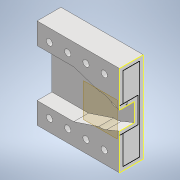
# Autodesk Inventor part: body
Saved by Autodesk Inventor 2022 (Build 260153000, 153)
## iProperties
Created: 2022-04-23
Part Number: body
Material: Generic
Document SubType Name: Modeling
Designer: efred
Density: 1 g/cm^3
Appearance: Default
Author: efred
Autodesk Inventor part; units mm, degrees
ref_plane "Work Plane1" through (0, 0, 0) normal (0, 0, 1) x (1, 0, 0)
sketch "Sketch1" plane through (0, 0, 0) normal (0, 0, 1) x (1, 0, 0)
  circle A0 centre (8, 0) radius 5 construction
  circle A1 centre (0, 18) radius 2 construction
  circle A2 centre (0, -18) radius 2 construction
  arc A3 (-10.2835, -9.5) -> (-3, -13.6748) centre (0, 0) ccw construction
  line L0 (-3, -13.6748) -> (-3, -18) construction
  arc A4 (-3, -18) -> (3, -18) centre (0, -18) ccw construction
  line L1 (3, -18) -> (3, -13.6748) construction
  arc A5 (3, -13.6748) -> (3, 13.6748) centre (0, 0) ccw construction
  line L2 (3, 13.6748) -> (3, 18) construction
  arc A6 (3, 18) -> (-3, 18) centre (0, 18) ccw construction
  line L3 (-3, 18) -> (-3, 13.6748) construction
  arc A7 (-3, 13.6748) -> (-10.2835, 9.5) centre (0, 0) ccw construction
  line L4 (-10.2835, 9.5) -> (-15.2835, 9.5) construction
  line L5 (-15.2835, 9.5) -> (-15.2835, -9.5) construction
  line L6 (-15.2835, -9.5) -> (-10.2835, -9.5) construction
  circle A8 centre (8, 0) radius 5.2
  circle A9 centre (0, -18) radius 1.7
  circle A10 centre (0, 18) radius 1.7
  line L7 (8, 0) -> (0, 0) construction
  line L8 (8, 0) -> (0, 0)
  line L9 (18.2, 24.7) -> (-6.7, 24.7)
  line L10 (-6.7, 24.7) -> (-6.7, -24.7)
  line L11 (-6.7, -24.7) -> (18.2, -24.7)
  line L12 (18.2, -24.7) -> (18.2, 24.7)
  point P0 (13.2, 0)
  point P1 (-1.7, 18)
  point P2 (0, 19.7)
  dimension "d0" = 0.2
  dimension "d3" = 5
  dimension "d4" = 5
  dimension "d5" = 5
  dimension "d20" = 3.4
  constraints: 12 end point, 3 equal length, 3 horizontal alignment, 2 centre point, 2 horizontal, 2 point on circle, 1 perpendicular, 1 vertical alignment, 4 other
  measures "d3" distance from line of point (13.2, 0) L12
  measures "d4" distance from line of L10 A10.start
  measures "d5" distance from line of A10.end L9
  measures "d20" diameter of A9
ref_plane "Work Plane2" through (3, -5, 1.9) normal (0, 0, 1) x (1, 0, 0)
ref_plane "Work Plane3" through (8, 0, 2) normal (0, 0, 1) x (1, 0, 0)
extrude "Extrusion1" add sketch "Sketch1" along normal up to surface (2 mm away)
sketch "Sketch2" plane through (-6.7, 24.7, 2) normal (0, 0, 1) x (1, 0, 0)
  circle A0 centre (6.7, -6.7) radius 1.7 projected
  circle A1 centre (6.7, -42.7) radius 1.7 projected
  circle A2 centre (14.7, -24.7) radius 5.2 construction
  line L0 (0, 0) -> (24.9, 0) projected
  line L1 (0, -49.4) -> (0, 0) projected
  line L2 (24.9, -49.4) -> (0, -49.4) projected
  line L3 (24.9, 0) -> (24.9, -49.4) projected
  circle A3 centre (14.7, -24.7) radius 2.5 construction
  circle A4 centre (14.7, -24.7) radius 2.7
  point P0 (6.7, -24.7)
  dimension "d8" = 0.2
  constraints: 1 centre point
  measures "d8" radial gap between concentric circles of A3 A4
ref_plane "Work Plane4" through (9.5, -2, 4.9) normal (0, 0, 1) x (1, 0, 0)
extrude "Extrusion2" add sketch "Sketch2" along normal up to surface (2.9 mm away)
sketch "Sketch3" plane through (-6.7, -24.7, 4.9) normal (0, 0, 1) x (1, 0, 0)
  arc A0 (18.0541, 25.7) -> (15.7, 28.0541) centre (14.7, 24.7) ccw construction
  line L0 (15.7, 33.0541) -> (15.7, 28.0541) construction
  line L1 (13.7, 33.0541) -> (15.7, 33.0541) construction
  line L2 (13.7, 28.0541) -> (13.7, 33.0541) construction
  arc A1 (13.7, 28.0541) -> (11.3459, 25.7) centre (14.7, 24.7) ccw construction
  line L3 (6.3459, 25.7) -> (11.3459, 25.7) construction
  line L4 (6.3459, 23.7) -> (6.3459, 25.7) construction
  line L5 (11.3459, 23.7) -> (6.3459, 23.7) construction
  arc A2 (11.3459, 23.7) -> (13.7, 21.3459) centre (14.7, 24.7) ccw construction
  line L6 (13.7, 16.3459) -> (13.7, 21.3459) construction
  line L7 (15.7, 16.3459) -> (13.7, 16.3459) construction
  line L8 (15.7, 21.3459) -> (15.7, 16.3459) construction
  arc A3 (15.7, 21.3459) -> (18.0541, 23.7) centre (14.7, 24.7) ccw construction
  line L9 (23.0541, 23.7) -> (18.0541, 23.7) construction
  line L10 (23.0541, 25.7) -> (23.0541, 23.7) construction
  line L11 (18.0541, 25.7) -> (23.0541, 25.7) construction
  circle A4 centre (14.7, 24.7) radius 8.4137 construction
  arc A5 (17.9486, 32.5696) -> (17.9486, 16.8304) centre (14.7, 24.7) ccw
  circle A6 centre (6.7, 42.7) radius 1.7 projected
  circle A7 centre (6.7, 6.7) radius 1.7 projected
  circle A8 centre (14.7, 24.7) radius 2.7 projected
  line L12 (0, 0) -> (0, 49.4) projected
  line L13 (24.9, 0) -> (0, 0) projected
  line L14 (24.9, 49.4) -> (24.9, 0) projected
  line L15 (0, 49.4) -> (24.9, 49.4) projected
  line L16 (0, 49.4) -> (0, 0) projected
  circle A9 centre (14.7, 24.7) radius 2.7 projected
  line L17 (14.7, 24.7) -> (0, 24.7) construction
  line L18 (17.9486, 16.8304) -> (24.9, 19.7)
  line L19 (24.9, 0) -> (24.9, 49.4) projected
  line L20 (17.9486, 32.5696) -> (24.9, 29.7)
  line L21 (13.7, 16.2452) -> (0, 11.7)
  line L22 (13.7, 33.1548) -> (0, 37.7)
  point P0 (6.7, 24.7)
  point P1 (0, 37.7)
  point P2 (24.9, 19.7)
  point P3 (0, 11.7)
  point P4 (0, 37.7)
  dimension "d11" = 0.1
  dimension "d13" = 10
  dimension "d17" = 5
  constraints: 10 end point, 3 point on circle, 3 point on line, 3 symmetric about line, 1 centre point, 1 coincident, 1 midpoint, 1 tangent, 1 vertical alignment, 4 other
  measures "d13" distance of L20.end L18.end
  measures "d17" vertical distance of L21.end A7.centre
ref_plane "Work Plane5" through (8, 0, 13.1) normal (0, 0, 1) x (-1, 0, 0)
ref_plane "Work Plane6" through (-0.3541, -8.3541, 13) normal (0, 0, 1) x (1, 0, 0)
extrude "Extrusion3" add sketch "Sketch3" along normal up to surface (8.1 mm away) contours A5 L22 L12 L15 L14 L20 | A5 L18 L14 L13 L12 L21
sketch "Sketch4" plane through (-6.7, -24.7, 0) normal (-1, 0, 0) x (0, 0, 1)
  line L0 (0, 49.4) -> (13, 49.4) projected
  line L1 (0, 49.4) -> (0, 0) projected
  line L2 (0, 0) -> (13, 0) projected
  line L3 (13, 0) -> (13, 11.7) projected
  line L4 (4.9, 11.7) -> (13, 11.7) projected
  line L5 (4.9, 11.7) -> (4.9, 37.7) projected
  line L6 (4.9, 37.7) -> (13, 37.7) projected
  line L7 (13, 37.7) -> (13, 49.4) projected
  point P0 (0, 24.7)
extrude "Extrusion4" add sketch "Sketch4" along normal blind 20
sketch "Sketch5" plane through (18.2, -24.7, 13) normal (0, 0, 1) x (1, 0, 0)
  circle A0 centre (-18.2, 6.7) radius 1.7 projected
  circle A1 centre (-18.2, 6.7) radius 1.7
  line L0 (0, 0) -> (-44.9, 0) projected
  circle A2 centre (-28.2, 6.7) radius 1.7
  circle A3 centre (-38.2, 6.7) radius 1.7
  circle A4 centre (-8.2, 6.7) radius 1.7
  circle A5 centre (-18.2, 6.7) radius 1.7
  circle A6 centre (-28.2, 6.7) radius 1.7
  point P0 (-18.2, 24.7)
  dimension "d23" = 10
  dimension "d26" = 10
  constraints: 6 centre point, 2 horizontal, 1 coincident, 1 concentric, 10 other
  measures "d23" distance of A1.centre A2.centre
  measures "d26" distance of A1.centre A4.centre
extrude "Extrusion5" cut sketch "Sketch5" against normal through all contours A2 | A3 | A4
mirror "Mirror1" about plane through (0, 0, 0) normal (0, 1, 0) of "Extrusion5"
sketch "Sketch6" plane through (18.2, -24.7, 0) normal (1, 0, 0) x (0, 0, -1)
  line L0 (0, 0) -> (-13, 0) projected
  line L1 (0, 0) -> (0, 49.4) projected
  line L2 (0, 49.4) -> (-13, 49.4) projected
  line L3 (-13, 49.4) -> (-13, 29.7) projected
  line L4 (-4.9, 29.7) -> (-13, 29.7) projected
  line L5 (-4.9, 29.7) -> (-4.9, 19.7) projected
  line L6 (-4.9, 19.7) -> (-13, 19.7) projected
  line L7 (-13, 19.7) -> (-13, 0) projected
  line L8 (-11, 31.7) -> (-11, 47.4)
  line L9 (-11, 47.4) -> (-2, 47.4)
  line L10 (-2, 47.4) -> (-2, 2)
  line L11 (-2, 2) -> (-11, 2)
  line L12 (-11, 2) -> (-11, 17.7)
  line L13 (-11, 17.7) -> (-2.9, 17.7)
  line L14 (-2.9, 17.7) -> (-2.9, 31.7)
  line L15 (-2.9, 31.7) -> (-11, 31.7)
  line L16 (-11, 31.7) -> (-13, 31.7)
  line L17 (-13, 49.4) -> (-13, 29.7) projected
  line L18 (-11, 17.7) -> (-13, 17.7)
  point P0 (0, 24.7)
  point P1 (-13, 31.7)
  dimension "d31" = 2
  constraints: 20 end point, 2 point on line, 1 horizontal, 1 perpendicular, 7 other
  measures "d31" distance between parallel lines of L4 L15
ref_plane "Work Plane7" through (36.9, -26.2379, 21.2621) normal (1, 0, 0) x (0, 0.9775, 0.2109)
extrude "Extrusion6" add sketch "Sketch6" along normal up to surface (18.7 mm away) contours L7 L6 L5 L4 L3 L16 L15 L14 L13 L18
body "Solid1"
